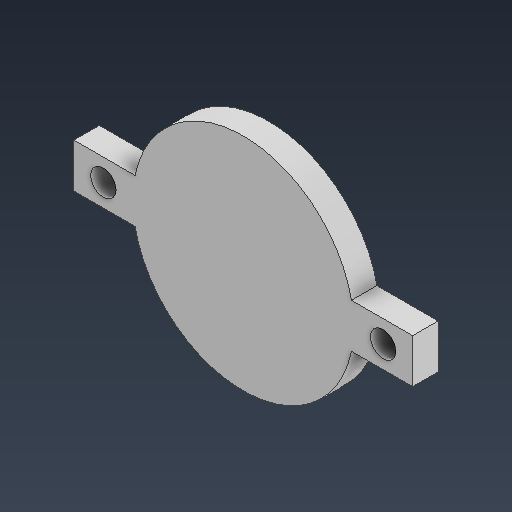
# Autodesk Inventor part: вт3
Saved by Autodesk Inventor 2025 (Build 290162000, 162)
## iProperties
Created: 2025-03-14
Part Number: вт3
Material: Типовые
Document SubType Name: Modeling
Designer: GameHD
Density: 1 g/cm^3
Appearance: По умолчанию
Author: GameHD
Autodesk Inventor part; units mm, degrees
ref_plane "YZ Plane" through (0, 0, 0) normal (1, 0, 0) x (0, 1, 0)
ref_plane "XZ Plane" through (0, 0, 0) normal (0, 1, 0) x (-1, 0, 0)
ref_plane "XY Plane" through (0, 0, 0) normal (0, 0, 1) x (1, 0, 0)
sketch "Эскиз1" plane through (0, 0, 0) normal (0, 0, 1) x (1, 0, 0)
  circle A0 centre (-15.0136, 0.7972) radius 1.5
  circle A1 centre (1.4615, 9.7972) radius 1.5
  arc A2 (2.9102, -8.5917) -> (0.0128, -8.5917) centre (1.4615, -8.2028) ccw
  line L0 (1.4615, 9.7972) -> (1.4615, -8.2028)
  circle A3 centre (17.9366, 0.7972) radius 1.5
  line L1 (-18.4887, -1.8013) -> (-11.5385, -1.8013)
  line L2 (-11.5385, -1.8013) -> (-11.5385, 3.3956)
  line L3 (-11.5385, 3.3956) -> (-18.4887, 3.3956)
  line L4 (-18.4887, 3.3956) -> (-18.4887, -1.8013)
  line L5 (-18.4887, -1.8013) -> (-11.5385, 3.3956) construction
  line L6 (-11.5385, -1.8013) -> (-18.4887, 3.3956) construction
  line L7 (-11.5385, 3.3956) -> (-10.2292, 3.3956)
  circle A4 centre (1.4615, 0.7972) radius 13
  circle A5 centre (1.4615, 0.7972) radius 9.5
  line L8 (-11.5385, -1.8013) -> (-10.8839, -1.8013)
  circle A6 centre (17.9366, 0.7972) radius 1.5
  line L9 (21.4117, -1.8013) -> (14.4615, -1.8013)
  line L10 (14.4615, -1.8013) -> (14.4615, 3.3956)
  line L11 (14.4615, 3.3956) -> (21.4117, 3.3956)
  line L12 (21.4117, 3.3956) -> (21.4117, -1.8013)
  line L13 (21.4117, -1.8013) -> (14.4615, 3.3956) construction
  line L14 (14.4615, -1.8013) -> (21.4117, 3.3956) construction
  line L15 (14.4615, 3.3956) -> (13.1521, 3.3956)
  line L16 (14.4615, -1.8013) -> (13.8068, -1.8013)
  point P0 (0, 0)
  point P1 (14.1991, 3.3956)
  point P2 (-11.2762, 3.3956)
  point P3 (-11.2762, -1.8013)
  point P4 (14.1991, -1.8013)
  dimension "d0" = 3
  constraints: 34 end point, 8 symmetric about line, 7 centre point, 2 horizontal, 2 midpoint, 2 parallel, 2 point on circle, 1 perpendicular, 1 vertical, 2 other
  measures "d0" diameter of A0
extrude "Выдавливание1" add sketch "Эскиз1" along normal blind 3 contours A1 A5 | A1 A5 A2 L0 | A5 A1 | L0 A2 A5 A1 | A2 A5 | L4 L3 L2 L1 | L2 A4 L8 | L2 L7 A4 | A4 | A4 L10 L16 | L15 L10 A4 | L10 L11 L12 L9
